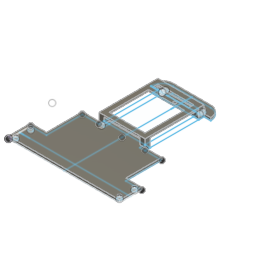
line follow car shape (Autodesk Fusion 360 design; units mm, degrees)
part number: 2026-01-10-19-25-23-777
Autodesk Fusion 360 part; units mm, degrees
sketch "Sketch1" plane through (0, 0, 0) normal (0, 1, 0) x (1, 0, 0)
  line L0 (0, 0) -> (130, 0)
  line L1 (130, 0) -> (130, 26)
  line L2 (0, 26) -> (0, 0)
  line L3 (0, 0) -> (0, 26)
  line L4 (0, 26) -> (18.5, 26)
  line L5 (18.5, 26) -> (18.5, 68)
  line L6 (65, 0) -> (65, 68)
  line L7 (130, 0) -> (130, 26)
  line L8 (130, 26) -> (111.5, 26)
  line L9 (111.5, 26) -> (111.5, 68)
  line L10 (0, 13) -> (130, 13)
  line L11 (92, 68) -> (92, 137)
  line L12 (92, 137) -> (38, 137)
  line L13 (38, 137) -> (38, 68)
  line L14 (44, 74) -> (86, 74)
  line L15 (86, 74) -> (86, 131)
  line L16 (86, 131) -> (44, 131)
  line L17 (44, 131) -> (44, 74)
  line L18 (111.5, 68) -> (92, 68)
  line L19 (38, 68) -> (18.5, 68)
  line L20 (65, 137) -> (100, 137)
  line L21 (65, 137) -> (30, 137)
  line L22 (87, 150) -> (43, 150)
  line L23 (30, 137) -> (50, 137)
  line L24 (100, 137) -> (80, 137)
  line L25 (80, 137) -> (80, 142)
  line L26 (80, 142) -> (50, 142)
  line L27 (50, 142) -> (50, 137)
  line L28 (30, 137) -> (41, 137)
  line L29 (30, 137) -> (45, 137)
  line L30 (41, 137) -> (43, 137)
  circle A0 centre (43, 141) radius 2
  line L31 (65, 68) -> (65, 150)
  circle A1 centre (87, 141) radius 2
  arc A2 (43, 150) -> (30, 137) centre (43, 137) ccw
  arc A3 (100, 137) -> (87, 150) centre (87, 137) ccw
  line L32 (0, 13) -> (11.5, 13)
  line L33 (0, 13) -> (4.2, 13)
  circle A4 centre (4.2, 21.8) radius 2.25
  circle A5 centre (4.2, 4.2) radius 2.25
  circle A6 centre (125.8, 21.8) radius 2.25
  circle A7 centre (125.8, 4.2) radius 2.25
  line L34 (65, 150) -> (65, 125.8)
  line L35 (86, 74) -> (92, 74)
  line L36 (38, 74) -> (44, 74)
  line L37 (86, 131) -> (92, 131)
  line L38 (44, 131) -> (38, 131)
  line L39 (41, 74) -> (41, 68)
  line L40 (41, 131) -> (41, 137)
  line L41 (38, 74) -> (44, 74)
  line L42 (44, 74) -> (44, 68)
  line L43 (44, 68) -> (38, 68)
  line L44 (38, 68) -> (38, 74)
  line L45 (86, 74) -> (92, 74)
  line L46 (92, 74) -> (92, 68)
  line L47 (92, 68) -> (86, 68)
  line L48 (86, 68) -> (86, 74)
  line L49 (38, 137) -> (44, 137)
  line L50 (44, 137) -> (44, 131)
  line L51 (44, 131) -> (38, 131)
  line L52 (38, 131) -> (38, 137)
  line L53 (92, 137) -> (86, 137)
  line L54 (86, 137) -> (86, 131)
  line L55 (86, 131) -> (92, 131)
  line L56 (92, 131) -> (92, 137)
  point P0 (111.5, 68)
  point P1 (130, 26)
  point P2 (18.5, 68)
  point P3 (0, 26)
  point P4 (-10.7147, 61.9143)
  point P5 (38, 68)
  point P6 (92, 68)
  point P7 (65, 68)
  dimension "d16" = 130
  dimension "d28" = 4
  dimension "d29" = 13
  dimension "d30" = 13
  dimension "d35" = 4.5
  dimension "d36" = 4.5
  dimension "d40" = 24.2
  constraint horizontal L0
  constraint vertical L1
  constraint horizontal L18
  constraint vertical L2
  constraint coincident L0.start L2.end
  constraint perpendicular L3 L4
  constraint perpendicular L5 L18
  constraint midpoint L0 L6.start
  constraint perpendicular L7 L8
  constraint perpendicular L9 L18
  constraint coincident P0 L9.end
  constraint coincident P1 L1.end
  constraint coincident P2 L5.end
  constraint coincident P3 L2.start
  constraint midpoint L3 L10.start
  constraint midpoint L7 L10.end
  constraint vertical L11
  constraint horizontal L12
  constraint vertical L13
  constraint coincident P5 L13.end
  constraint coincident P7 L6.end
  constraint collinear L18 L19
  constraint midpoint L12 L20.start
  constraint parallel L12 L20
  constraint parallel L12 L21
  constraint coincident L12 L23.end
  constraint coincident L12 L24.end
  constraint perpendicular L24 L25
  constraint perpendicular L25 L26
  constraint perpendicular L12 L27
  constraint coincident L21 L29.end
  constraint parallel L12 L30
  constraint perpendicular L26 L31
  constraint symmetric A0 L31 A1
  constraint tangent L22 A2
  constraint coincident L21.end L23.start
  constraint tangent L22 A3
  constraint coincident L20.end L24.start
  constraint coincident L10 L32.end
  constraint perpendicular L2 L32
  constraint coincident L10 L33.end
  constraint symmetric L6 A4 A6
  constraint symmetric L6 A5 A7
  constraint coincident L31 L34.end
  constraint perpendicular L16 L34
  constraint coincident L11 L35.end
  constraint perpendicular L11 L35
  constraint coincident L13 L36.start
  constraint perpendicular L17 L36
  constraint coincident L11 L37.end
  constraint perpendicular L11 L37
  constraint coincident L13 L38.end
  constraint perpendicular L13 L38
  constraint midpoint L36 L39.start
  constraint perpendicular L36 L39
  constraint midpoint L38 L40.start
  constraint horizontal L41
  constraint vertical L42
  constraint horizontal L43
  constraint vertical L44
  constraint horizontal L45
  constraint vertical L46
  constraint horizontal L47
  constraint vertical L48
  constraint coincident P6 L11.start
  constraint horizontal L49
  constraint vertical L50
  constraint horizontal L51
  constraint vertical L52
  constraint horizontal L53
  constraint vertical L54
  constraint horizontal L55
  constraint vertical L56
  measures "d16" distance of L0.start L0.end
  measures "d28" diameter of A0
  measures "d29" radius of A2
  measures "d30" radius of A3
  measures "d35" diameter of A4
  measures "d36" diameter of A5
  measures "d40" distance of L31.end L34.end
extrude "Extrude3" add sketch "Sketch1" along normal blind 3 contours L0 L2 L3 L6 L10 L32 L33 | L0 L1 L6 L7 L10 | L2 L3 L4 L5 L6 L10 L14 L19 L31 L32 L33 L42 L43 | L1 L6 L7 L8 L9 L10 L14 L18 L31 L47 L48 | L36 L39 L41 L42 L43 | L11 L35 L45 L46 L47 L48 | L13 L36 L39 L41 L43 L44 | L12 L16 L21 L23 L29 L31 L34 L50 | L12 L21 L23 L29 L30 L38 L40 L49 L50 L51 | L11 L12 L20 L24 L37 L53 L54 L55 L56 | L12 L16 L20 L24 L31 L34 L54 | L12 L13 L21 L23 L28 L29 L38 L40 L49 L51 L52 | L12 L21 L22 L23 L26 L27 L28 L29 L30 L31 A2 L34 L49 | L12 L20 L22 L24 L25 L26 L31 A3 L34 L53 makes body 1 at (70, 0, -147.3333) makes body 2 at (74, 0, -40)
sketch "Sketch3" plane through (0, 3, 0) normal (0, 1, 0) x (-1, 0, 0)
  circle A0 centre (-125.8, -4.2) radius 2.25
  circle A1 centre (-4.2, -21.8) radius 2.25
  circle A2 centre (-4.2, -4.2) radius 2.25
  circle A3 centre (-125.8, -21.8) radius 2.25
  line L0 (-38, -68) -> (-18.5, -68)
  line L1 (-18.5, -68) -> (-18.5, -26)
  line L2 (-18.5, -26) -> (0, -26)
  line L3 (0, -26) -> (0, 0)
  line L4 (0, 0) -> (-130, 0)
  line L5 (-130, 0) -> (-130, -26)
  line L6 (-130, -26) -> (-111.5, -26)
  line L7 (-111.5, -26) -> (-111.5, -68)
  line L8 (-111.5, -68) -> (-92, -68)
  line L9 (-92, -68) -> (-92, -74)
  line L10 (-92, -74) -> (-38, -74)
  line L11 (-38, -74) -> (-38, -68)
  line L12 (-38, -74) -> (-44, -74)
  line L13 (-44, -74) -> (-44, -68)
  line L14 (-44, -68) -> (-38, -68)
  line L15 (-38, -68) -> (-38, -74)
  line L16 (-92, -74) -> (-86, -74)
  line L17 (-86, -74) -> (-86, -68)
  line L18 (-86, -68) -> (-92, -68)
  line L19 (-92, -68) -> (-92, -74)
  line L20 (-38, -137) -> (-44, -137)
  line L21 (-44, -137) -> (-44, -131)
  line L22 (-44, -131) -> (-38, -131)
  line L23 (-38, -131) -> (-38, -137)
  line L24 (-92, -137) -> (-86, -137)
  line L25 (-86, -137) -> (-86, -131)
  line L26 (-86, -131) -> (-92, -131)
  line L27 (-92, -131) -> (-92, -137)
  constraint horizontal L12
  constraint vertical L13
  constraint horizontal L14
  constraint vertical L15
  constraint coincident L10.end L11.start
  constraint horizontal L16
  constraint vertical L17
  constraint horizontal L18
  constraint vertical L19
  constraint coincident L9.end L10.start
  constraint horizontal L20
  constraint vertical L21
  constraint horizontal L22
  constraint vertical L23
  constraint horizontal L24
  constraint vertical L25
  constraint horizontal L26
  constraint vertical L27
sketch "Sketch4" plane through (0, 10, 0) normal (0, 1, 0) x (-1, 0, 0)
  line L0 (-38, -137) -> (-92, -137)
  line L1 (-92, -137) -> (-92, -68)
  line L2 (-92, -68) -> (-38, -68)
  line L3 (-38, -68) -> (-38, -137)
  line L4 (-44, -131) -> (-86, -131)
  line L5 (-86, -131) -> (-86, -74)
  line L6 (-86, -74) -> (-44, -74)
  line L7 (-44, -74) -> (-44, -131)
  line L8 (-44, -125) -> (-44, -120)
  line L9 (-86, -120) -> (-44, -120)
  line L10 (-44, -125) -> (-86, -125)
  line L11 (-65, -122.5) -> (-72.5, -122.5)
  circle A0 centre (-72.5, -122.5) radius 1.75
  line L12 (-65, -68) -> (-65, -150)
  circle A1 centre (-57.5, -122.5) radius 1.75
  line L13 (-38, -137) -> (-38, -131)
  line L14 (-38, -131) -> (-44, -131)
  line L15 (-44, -131) -> (-44, -137)
  line L16 (-44, -137) -> (-38, -137)
  line L17 (-38, -74) -> (-38, -68)
  line L18 (-38, -68) -> (-44, -68)
  line L19 (-44, -68) -> (-44, -74)
  line L20 (-44, -74) -> (-38, -74)
  line L21 (-92, -137) -> (-86, -137)
  line L22 (-86, -137) -> (-86, -131)
  line L23 (-86, -131) -> (-92, -131)
  line L24 (-92, -131) -> (-92, -137)
  line L25 (-92, -74.1066) -> (-86, -74.1066)
  line L26 (-86, -74.1066) -> (-86, -68)
  line L27 (-86, -68) -> (-92, -68)
  line L28 (-92, -68) -> (-92, -74.1066)
  dimension "d51" = 7.5
  dimension "d52" = 3.5
  constraint horizontal L0
  constraint vertical L1
  constraint horizontal L2
  constraint vertical L3
  constraint horizontal L4
  constraint vertical L5
  constraint horizontal L6
  constraint vertical L7
  constraint coincident L7 L8.start
  constraint coincident L7 L8.end
  constraint coincident L5 L9.start
  constraint perpendicular L7 L9
  constraint coincident L5 L10.end
  constraint perpendicular L5 L10
  constraint parallel L9 L11
  constraint coincident L11.end A0.centre
  constraint symmetric A0 L12 A1
  constraint horizontal L21
  constraint vertical L22
  constraint horizontal L23
  constraint vertical L24
  constraint horizontal L25
  constraint vertical L26
  constraint horizontal L27
  constraint vertical L28
  constraint coincident L2 L26.end
  constraint coincident L1 L25.start
  measures "d51" distance of L11.start L11.end
  measures "d52" diameter of A0
sketch "Sketch5" plane through (0, 3, 0) normal (0, 1, 0) x (-1, 0, 0)
  line L0 (-92, -74) -> (-86, -74)
  line L1 (-86, -74) -> (-86, -69)
  line L2 (-92, -69) -> (-92, -74)
  line L3 (-92, -68) -> (-86, -68)
  line L4 (-86, -68) -> (-86, -74)
  line L5 (-86, -74) -> (-92, -74)
  line L6 (-92, -74) -> (-92, -68)
  constraint horizontal L0
  constraint vertical L1
  constraint vertical L2
  constraint horizontal L3
  constraint vertical L4
  constraint horizontal L5
  constraint vertical L6
extrude "Extrude11" add sketch "Sketch3" along normal blind 8 contours L10 L11 L12 L13 L14 L15 | L9 L10 L16 L17 L18 L19 | L20 L21 L22 L23 | L24 L25 L26 L27 bodies 1 2
extrude "Extrude12" add sketch "Sketch4" along normal blind 2 contours L0 L3 L13 L14 L15 L16 | L0 L4 L12 L15 | L3 L7 L8 L14 L20 | L0 L4 L12 L22 | L2 L3 L17 L18 L19 L20 | L0 L1 L21 L22 L23 L24 | L7 L8 L9 L10 L12 | L2 L6 L12 L19 | L1 L5 L23 L25 | L5 L9 L10 L12 | L2 L6 L12 L26 | L1 L2 L5 L25 L26 L27 L28 bodies 1 2
